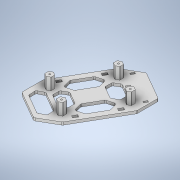
# Autodesk Inventor part: top_body
Saved by Autodesk Inventor 2022 (Build 260153000, 153)
## iProperties
Created: 2022-01-21
Part Number: top_body
Material: Generic
Document SubType Name: Modeling
Designer: felix
Density: 1 g/cm^3
Appearance: Default
Author: felix
Autodesk Inventor part; units mm, degrees
ref_plane "YZ Plane" through (0, 0, 0) normal (1, 0, 0) x (0, 1, 0)
ref_plane "XZ Plane" through (0, 0, 0) normal (0, 1, 0) x (-1, 0, 0)
ref_plane "XY Plane" through (0, 0, 0) normal (0, 0, 1) x (1, 0, 0)
sketch "Sketch1" plane through (0, 0, 0) normal (0, 1, 0) x (-1, 0, 0)
  line L0 (-6.75, 41.286) -> (6.75, 41.286)
  line L1 (-8.75, 41.286) -> (-12.4595, 41.286)
  line L2 (10.832, 42.286) -> (27.4333, 71.0403)
  line L3 (39.1324, 45.1163) -> (-87.7037, 118.3452) construction
  line L4 (27.4333, 73.0403) -> (16.6536, 91.7113)
  line L5 (-8.3049, 49.4102) -> (11.6951, 84.0512) construction
  line L6 (11.6951, 84.0512) -> (-40.2664, 114.0512) construction
  line L7 (-40.2664, 114.0512) -> (-60.2664, 79.4102) construction
  line L8 (-60.2664, 79.4102) -> (-8.3049, 49.4102) construction
  line L9 (27.4333, 73.0403) -> (16.6536, 91.7113)
  line L10 (-13.4595, 41.554) -> (-38.9761, 56.286)
  line L11 (15.9215, 92.4434) -> (-9.5951, 107.1754)
  line L12 (-38.9761, 56.286) -> (-9.5951, 107.1754) construction
  line L13 (8.75, 41.286) -> (9.0999, 41.286)
  line L14 (6.75, 41.286) -> (8.75, 41.286)
  line L15 (-6.75, 41.286) -> (-8.75, 41.286)
  line L16 (-68.0796, 76.6947) -> (-74.8296, 88.386)
  line L17 (-67.0796, 74.9626) -> (-65.2248, 71.7501)
  line L18 (-76.0045, 92.4211) -> (-59.413, 121.1585)
  line L19 (-57.6825, 122.1585) -> (-36.1133, 122.1754)
  line L20 (-57.6825, 122.1585) -> (-36.1133, 122.1754)
  line L21 (-64.4928, 71.0181) -> (-38.9761, 56.286)
  line L22 (-35.1118, 121.9075) -> (-9.5951, 107.1754)
  line L23 (-75.8296, 90.1181) -> (-76.0045, 90.4211)
  line L24 (-74.8296, 88.386) -> (-75.8296, 90.1181)
  line L25 (-68.0796, 76.6947) -> (-67.0796, 74.9626)
  line L26 (-41.8469, 122.123) -> (-39.8469, 122.123)
  line L27 (8.342, 47.7751) -> (2.3676, 47.4271)
  line L28 (0.464, 48.5261) -> (-2.2218, 53.8742)
  line L29 (-2.1666, 55.7718) -> (9.255, 75.5546)
  line L30 (10.8707, 76.5512) -> (16.8452, 76.8992)
  line L31 (18.7488, 75.8002) -> (21.4346, 70.4522)
  line L32 (21.3794, 68.5546) -> (9.9577, 48.7718)
  line L33 (-53.2274, 80.0021) -> (-54.9595, 77.0021)
  line L34 (-55.3925, 76.7521) -> (-58.8566, 76.7521)
  line L35 (-59.2896, 77.0021) -> (-61.0216, 80.0021)
  line L36 (-61.0216, 80.5021) -> (-59.2896, 83.5021)
  line L37 (-58.8566, 83.7521) -> (-55.3925, 83.7521)
  line L38 (-54.9595, 83.5021) -> (-53.2274, 80.5021)
  circle A0 centre (-57.1245, 80.2521) radius 0.9
  line L39 (-37.2595, 107.6594) -> (-35.5274, 110.6594)
  line L40 (-35.5274, 111.1594) -> (-37.2595, 114.1594)
  line L41 (-37.6925, 114.4094) -> (-41.1566, 114.4094)
  line L42 (-41.5896, 114.1594) -> (-43.3216, 111.1594)
  line L43 (-43.3216, 110.6594) -> (-41.5896, 107.6594)
  line L44 (-41.1566, 107.4094) -> (-37.6925, 107.4094)
  circle A1 centre (-39.4245, 110.9094) radius 0.9
  line L45 (-11.3118, 55.8021) -> (-13.0438, 52.8021)
  line L46 (-13.0438, 52.3021) -> (-11.3118, 49.3021)
  line L47 (-10.8788, 49.0521) -> (-7.4147, 49.0521)
  line L48 (-6.9816, 49.3021) -> (-5.2496, 52.3021)
  line L49 (-5.2496, 52.8021) -> (-6.9816, 55.8021)
  line L50 (-7.4147, 56.0521) -> (-10.8788, 56.0521)
  circle A2 centre (-9.1467, 52.5521) radius 0.9
  line L51 (10.7184, 86.4594) -> (12.4504, 83.4594)
  line L52 (6.8212, 86.7094) -> (10.2853, 86.7094)
  line L53 (4.6562, 83.4594) -> (6.3882, 86.4594)
  circle A3 centre (8.5533, 83.2094) radius 0.9
  line L54 (12.4504, 82.9594) -> (10.7184, 79.9594)
  line L55 (10.2853, 79.7094) -> (6.8212, 79.7094)
  line L56 (6.3882, 79.9594) -> (4.6562, 82.9594)
  line L57 (-55.4722, 69.7141) -> (-53.9722, 72.3121)
  line L58 (-53.9722, 72.3121) -> (-49.642, 69.8121)
  line L59 (-49.642, 69.8121) -> (-51.142, 67.2141)
  line L60 (-51.142, 67.2141) -> (-55.4722, 69.7141)
  line L61 (-29.4722, 114.7474) -> (-30.9722, 112.1493)
  line L62 (-30.9722, 112.1493) -> (-26.642, 109.6493)
  line L63 (-26.642, 109.6493) -> (-25.142, 112.2474)
  line L64 (-25.142, 112.2474) -> (-29.4722, 114.7474)
  line L65 (-19.0991, 48.7141) -> (-17.5991, 51.3121)
  line L66 (-17.5991, 51.3121) -> (-21.9292, 53.8121)
  line L67 (-21.9292, 53.8121) -> (-23.4292, 51.2141)
  line L68 (-23.4292, 51.2141) -> (-19.0991, 48.7141)
  line L69 (2.5708, 96.2474) -> (6.9009, 93.7474)
  line L70 (1.0708, 93.6493) -> (2.5708, 96.2474)
  line L71 (5.4009, 91.1493) -> (1.0708, 93.6493)
  line L72 (6.9009, 93.7474) -> (5.4009, 91.1493)
  line L73 (-46.6809, 74.1125) -> (-44.8508, 67.2824)
  line L74 (-43.9189, 66.068) -> (-28.0333, 56.8964)
  line L75 (-26.5157, 56.6966) -> (-19.6855, 58.5267)
  line L76 (-18.2713, 60.9762) -> (-20.1015, 67.8063)
  line L77 (-21.0333, 69.0207) -> (-36.9189, 78.1923)
  line L78 (-38.4366, 78.3921) -> (-45.2667, 76.562)
  line L79 (18.1584, 76.9758) -> (1.0543, 47.3506) construction
  line L80 (-47.6364, 61.286) -> (-30.8723, 90.3222) construction
  line L81 (-30.3159, 51.286) -> (-13.5518, 80.3222) construction
  line L82 (12.8814, 45.8357) -> (-2.7058, 54.8379) construction
  line L83 (25.3698, 67.436) -> (9.8848, 76.3791) construction
  line L84 (-28.8857, 104.9347) -> (-22.0556, 106.7649)
  line L85 (-20.5379, 106.5651) -> (-4.6523, 97.3935)
  line L86 (-3.7204, 96.1791) -> (-1.8903, 89.3489)
  line L87 (-3.3045, 86.8995) -> (-10.1347, 85.0693)
  line L88 (-11.6523, 85.2691) -> (-27.5379, 94.4407)
  line L89 (-28.4698, 95.6551) -> (-30.2999, 102.4852)
  line L90 (-18.2554, 112.1754) -> (-35.0194, 83.1393) construction
  line L91 (-0.9349, 102.1754) -> (-17.6989, 73.1393) construction
  line L92 (-57.1245, 80.2521) -> (8.5533, 83.2094) construction
  line L93 (-9.1467, 52.5521) -> (-39.4245, 110.9094) construction
  line L94 (-17.7537, 59.0444) -> (-47.1986, 76.0444) construction
  line L95 (-1.3727, 87.4171) -> (-30.8175, 104.4171) construction
  line L96 (-52.6513, 88.8701) -> (-40.527, 81.8701) construction
  line L97 (-44.6513, 102.7265) -> (-32.527, 95.7265) construction
  line L98 (-36.6202, 102.6368) -> (-48.5581, 81.9597) construction
  line L99 (3.4953, 73.5784) -> (-3.3351, 61.7479)
  line L100 (-5.0895, 60.748) -> (-10.826, 60.8121)
  line L101 (-12.5244, 61.7927) -> (-15.4482, 66.7286)
  line L102 (-15.4595, 68.7479) -> (-8.6291, 80.5784)
  line L103 (-6.8747, 81.5783) -> (-1.1382, 81.5143)
  line L104 (0.5603, 80.5337) -> (3.484, 75.5977)
  line L105 (-3.9199, 60.735) -> (-16.0443, 67.735) construction
  line L106 (4.0801, 74.5914) -> (-8.0443, 81.5914) construction
  line L107 (-0.0131, 81.5017) -> (-11.951, 60.8247) construction
  arc A4 (-57.6825, 122.1585) -> (-59.413, 121.1585) centre (-57.681, 120.1585) ccw
  arc A5 (-76.0045, 92.4211) -> (-76.0045, 90.4211) centre (-74.2725, 91.4211) ccw
  arc A6 (-35.1118, 121.9075) -> (-36.1133, 122.1754) centre (-36.1118, 120.1754) ccw
  arc A7 (16.6536, 91.7113) -> (15.9215, 92.4434) centre (14.9215, 90.7113) ccw
  arc A8 (27.4333, 71.0403) -> (27.4333, 73.0403) centre (25.7012, 72.0403) ccw
  arc A9 (9.0999, 41.286) -> (10.832, 42.286) centre (9.0999, 43.286) ccw
  arc A10 (-13.4595, 41.554) -> (-12.4595, 41.286) centre (-12.4595, 43.286) ccw
  arc A11 (-65.2248, 71.7501) -> (-64.4928, 71.0181) centre (-63.4928, 72.7501) ccw
  arc A12 (-61.0216, 80.5021) -> (-61.0216, 80.0021) centre (-60.5886, 80.2521) ccw
  arc A13 (-58.8566, 83.7521) -> (-59.2896, 83.5021) centre (-58.8566, 83.2521) ccw
  arc A14 (-54.9595, 83.5021) -> (-55.3925, 83.7521) centre (-55.3925, 83.2521) ccw
  arc A15 (-53.2274, 80.0021) -> (-53.2274, 80.5021) centre (-53.6604, 80.2521) ccw
  arc A16 (-55.3925, 76.7521) -> (-54.9595, 77.0021) centre (-55.3925, 77.2521) ccw
  arc A17 (-59.2896, 77.0021) -> (-58.8566, 76.7521) centre (-58.8566, 77.2521) ccw
  arc A18 (-43.3216, 111.1594) -> (-43.3216, 110.6594) centre (-42.8886, 110.9094) ccw
  arc A19 (-41.1566, 114.4094) -> (-41.5896, 114.1594) centre (-41.1566, 113.9094) ccw
  arc A20 (-37.2595, 114.1594) -> (-37.6925, 114.4094) centre (-37.6925, 113.9094) ccw
  arc A21 (-35.5274, 110.6594) -> (-35.5274, 111.1594) centre (-35.9604, 110.9094) ccw
  arc A22 (-37.6925, 107.4094) -> (-37.2595, 107.6594) centre (-37.6925, 107.9094) ccw
  arc A23 (-41.5896, 107.6594) -> (-41.1566, 107.4094) centre (-41.1566, 107.9094) ccw
  arc A24 (6.8212, 86.7094) -> (6.3882, 86.4594) centre (6.8212, 86.2094) ccw
  arc A25 (10.7184, 86.4594) -> (10.2853, 86.7094) centre (10.2853, 86.2094) ccw
  arc A26 (12.4504, 82.9594) -> (12.4504, 83.4594) centre (12.0174, 83.2094) ccw
  arc A27 (10.2853, 79.7094) -> (10.7184, 79.9594) centre (10.2853, 80.2094) ccw
  arc A28 (6.3882, 79.9594) -> (6.8212, 79.7094) centre (6.8212, 80.2094) ccw
  arc A29 (4.6562, 83.4594) -> (4.6562, 82.9594) centre (5.0892, 83.2094) ccw
  arc A30 (-13.0438, 52.8021) -> (-13.0438, 52.3021) centre (-12.6108, 52.5521) ccw
  arc A31 (-11.3118, 49.3021) -> (-10.8788, 49.0521) centre (-10.8788, 49.5521) ccw
  arc A32 (-7.4147, 49.0521) -> (-6.9816, 49.3021) centre (-7.4147, 49.5521) ccw
  arc A33 (-5.2496, 52.3021) -> (-5.2496, 52.8021) centre (-5.6826, 52.5521) ccw
  arc A34 (-6.9816, 55.8021) -> (-7.4147, 56.0521) centre (-7.4147, 55.5521) ccw
  arc A35 (-10.8788, 56.0521) -> (-11.3118, 55.8021) centre (-10.8788, 55.5521) ccw
  arc A36 (-45.2667, 76.562) -> (-46.6809, 74.1125) centre (-44.7491, 74.6301) ccw
  arc A37 (-36.9189, 78.1923) -> (-38.4366, 78.3921) centre (-37.9189, 76.4603) ccw
  arc A38 (-44.8508, 67.2824) -> (-43.9189, 66.068) centre (-42.9189, 67.8) ccw
  arc A39 (-28.0333, 56.8964) -> (-26.5157, 56.6966) centre (-27.0333, 58.6284) ccw
  arc A40 (-19.6855, 58.5267) -> (-18.2713, 60.9762) centre (-20.2032, 60.4586) ccw
  arc A41 (-20.1015, 67.8063) -> (-21.0333, 69.0207) centre (-22.0333, 67.2887) ccw
  arc A42 (-28.4698, 95.6551) -> (-27.5379, 94.4407) centre (-26.5379, 96.1728) ccw
  arc A43 (-28.8857, 104.9347) -> (-30.2999, 102.4852) centre (-28.3681, 103.0029) ccw
  arc A44 (-20.5379, 106.5651) -> (-22.0556, 106.7649) centre (-21.5379, 104.833) ccw
  arc A45 (-3.7204, 96.1791) -> (-4.6523, 97.3935) centre (-5.6523, 95.6614) ccw
  arc A46 (-3.3045, 86.8995) -> (-1.8903, 89.3489) centre (-3.8222, 88.8313) ccw
  arc A47 (-11.6523, 85.2691) -> (-10.1347, 85.0693) centre (-10.6523, 87.0012) ccw
  arc A48 (-2.1666, 55.7718) -> (-2.2218, 53.8742) centre (-0.4346, 54.7718) ccw
  arc A49 (10.8707, 76.5512) -> (9.255, 75.5546) centre (10.9871, 74.5546) ccw
  arc A50 (18.7488, 75.8002) -> (16.8452, 76.8992) centre (16.9615, 74.9026) ccw
  arc A51 (21.3794, 68.5546) -> (21.4346, 70.4522) centre (19.6473, 69.5546) ccw
  arc A52 (8.342, 47.7751) -> (9.9577, 48.7718) centre (8.2257, 49.7718) ccw
  arc A53 (0.464, 48.5261) -> (2.3676, 47.4271) centre (2.2512, 49.4237) ccw
  arc A54 (-15.4595, 68.7479) -> (-15.4482, 66.7286) centre (-13.7274, 67.7479) ccw
  arc A55 (-6.8747, 81.5783) -> (-8.6291, 80.5784) centre (-6.897, 79.5784) ccw
  arc A56 (0.5603, 80.5337) -> (-1.1382, 81.5143) centre (-1.1605, 79.5144) ccw
  arc A57 (3.4953, 73.5784) -> (3.484, 75.5977) centre (1.7632, 74.5784) ccw
  arc A58 (-5.0895, 60.748) -> (-3.3351, 61.7479) centre (-5.0671, 62.7479) ccw
  arc A59 (-12.5244, 61.7927) -> (-10.826, 60.8121) centre (-10.8037, 62.812) ccw
  line L108 (-45.2361, 101.7135) -> (-52.0665, 89.883)
  line L109 (-52.0552, 87.8637) -> (-49.1315, 82.9278)
  line L110 (-47.433, 81.9472) -> (-41.6965, 81.8831)
  line L111 (-37.7452, 102.6494) -> (-43.4818, 102.7134)
  line L112 (-33.1231, 96.7328) -> (-36.0468, 101.6688)
  line L113 (-39.9421, 82.883) -> (-33.1118, 94.7135)
  arc A60 (-41.6965, 81.8831) -> (-39.9421, 82.883) centre (-41.6742, 83.883) ccw
  arc A61 (-33.1118, 94.7135) -> (-33.1231, 96.7328) centre (-34.8438, 95.7135) ccw
  arc A62 (-36.0468, 101.6688) -> (-37.7452, 102.6494) centre (-37.7676, 100.6495) ccw
  arc A63 (-43.4818, 102.7134) -> (-45.2361, 101.7135) centre (-43.5041, 100.7135) ccw
  arc A64 (-52.0665, 89.883) -> (-52.0552, 87.8637) centre (-50.3345, 88.883) ccw
  arc A65 (-49.1315, 82.9278) -> (-47.433, 81.9472) centre (-47.4107, 83.9471) ccw
  point P0 (10.2546, 41.286)
  point P1 (-12.9954, 41.286)
  point P2 (28.0107, 72.0403)
  point P3 (19.1326, 56.6632)
  point P4 (-67.7039, 106.7983)
  point P5 (-8.3049, 49.4102)
  point P6 (-24.2856, 81.7307)
  point P7 (9.4185, 47.8379)
  point P8 (21.9185, 69.4885)
  point P9 (-53.0831, 80.2521)
  point P10 (-55.1038, 76.7521)
  point P11 (-59.1452, 76.7521)
  point P12 (-61.166, 80.2521)
  point P13 (-59.1452, 83.7521)
  point P14 (-55.1038, 83.7521)
  point P15 (-37.4038, 107.4094)
  point P16 (-35.3831, 110.9094)
  point P17 (-37.4038, 114.4094)
  point P18 (-41.4452, 114.4094)
  point P19 (-43.466, 110.9094)
  point P20 (-41.4452, 107.4094)
  point P21 (-11.1674, 56.0521)
  point P22 (-13.1882, 52.5521)
  point P23 (-11.1674, 49.0521)
  point P24 (-7.126, 49.0521)
  point P25 (-5.1053, 52.5521)
  point P26 (-7.126, 56.0521)
  point P27 (10.574, 86.7094)
  point P28 (12.5947, 83.2094)
  point P29 (6.5326, 86.7094)
  point P30 (4.5118, 83.2094)
  point P31 (10.574, 79.7094)
  point P32 (6.5326, 79.7094)
  point P33 (-44.6364, 66.4822)
  point P34 (-27.3159, 56.4822)
  point P35 (-20.3159, 68.6065)
  point P36 (-37.6364, 78.6065)
  point P37 (-21.2554, 106.9793)
  point P38 (-3.9349, 96.9793)
  point P39 (-10.9349, 84.8549)
  point P40 (-28.2554, 94.8549)
  point P41 (8.5533, 83.2094)
  dimension "d82" = 23.25
  dimension "d88" = 120
  dimension "d89" = 120
  dimension "d90" = 35.512
  dimension "d91" = 17.756
  dimension "d92" = 17.756
  dimension "d95" = 40
  dimension "d97" = 20
  dimension "d99" = 30
  dimension "d102" = 60
  dimension "d145" = 180
  dimension "d146" = 30
  dimension "d147" = 8.1242
  dimension "d148" = 8.1242
  dimension "d155" = 1.8
  dimension "d156" = 7
  dimension "d157" = 1.4
  dimension "d158" = 1.4
  dimension "d160" = 3
  dimension "d162" = 3
  dimension "d163" = 9
  dimension "d169" = 6
  dimension "d170" = 10
  dimension "d171" = 20
  dimension "d172" = 14
  dimension "d179" = 7
  dimension "d181" = 2
  dimension "d186" = 0.5
  dimension "d187" = 0.5
  dimension "d189" = 2
  dimension "d190" = 2
  dimension "d191" = 4
  dimension "d192" = 16
  dimension "d193" = 8
  dimension "d194" = 14
  dimension "d195" = 8
  dimension "d204" = 14
  dimension "d206" = 18.762
  dimension "d207" = 28.2702
  dimension "d238" = 5
  dimension "d244" = 25
  dimension "d245" = 12.5
  dimension "d246" = 0
  dimension "d247" = 4
  constraints: 228 end point, 124 point on circle, 112 tangent, 110 point on line, 79 symmetric about line, 66 centre point, 51 equal radius, 16 parallel, 9 equal length, 6 perpendicular, 4 collinear, 3 coincident, 3 midpoint, 2 horizontal, 22 other
  measures "d82" distance of point (10.255, 41.286) point (-12.995, 41.286)
  measures "d88" angle of L2 L1
  measures "d89" angle of L4 L2
  measures "d90" distance of point (10.255, 41.286) point (28.011, 72.04)
  measures "d91" distance of point (19.133, 56.663) point (10.255, 41.286)
  measures "d92" distance of point (28.011, 72.04) point (19.133, 56.663)
  measures "d95" distance of L5.start L5.end
  measures "d97" distance from line of L3 L5.start
  measures "d99" distance of L10.end point (-12.995, 41.286)
  measures "d102" distance of L7.end L5.start
  measures "d145" angle of L10 L21
  measures "d146" distance from line of L5 point (-24.286, 81.731)
  measures "d147" distance from line of L0 L5.start
  measures "d148" distance from line of L4 L5.end
  measures "d155" diameter of A0
  measures "d156" distance between parallel lines of L38 L35
  measures "d157" distance edge to line of A0 L7
  measures "d158" distance edge to line of A0 L8
  measures "d160" distance between parallel lines of L58 L60
  measures "d162" distance between parallel lines of L8 L58
  measures "d163" distance between parallel lines of L57 L7
  measures "d169" distance between parallel lines of L21 L74
  measures "d170" distance from line of L12 point (-27.316, 56.482)
  measures "d171" distance of point (-44.636, 66.482) point (-27.316, 56.482)
  measures "d172" distance between parallel lines of L77 L74
  measures "d179" distance from line of L94.end L80
  measures "d181" radius of A4
  measures "d186" radius of A12
  measures "d187" radius of A27
  measures "d189" radius of A36
  measures "d190" radius of A54
  measures "d191" distance between parallel lines of L29 L99
  measures "d192" distance of L105.start L106.start
  measures "d193" distance from line of L3 L106.start
  measures "d194" distance between parallel lines of L99 L102
  measures "d195" distance between parallel lines of L106 L3
  measures "d204" distance between parallel lines of L32 L29
  measures "d206" distance between parallel lines of L88 L77
  measures "d207" distance between parallel lines of L113 L102
  measures "d238" distance of L59.end L57.start
  measures "d244" distance of point (21.919, 69.488) point (9.419, 47.838)
  measures "d245" distance from line of L3 point (9.419, 47.838)
  measures "d246" angle of L83 L82
  measures "d247" distance between parallel lines of L2 L32
extrude "Extrusion1_main_body" add sketch "Sketch1" along normal blind 3 contours L15 L1 A10 L10 L21 A11 L17 L25 L16 L24 L23 A5 L18 A4 L19 A6 L22 L11 A7 L4 A8 L2 A9 L13 L14 L0
extrude "Extrusion2_main_body" add sketch "Sketch1" along normal blind 16 contours L33 A16 L34 A17 L35 A12 L36 A13 L37 A14 L38 A15 | A22 L44 A23 L43 A18 L42 A19 L41 A20 L40 A21 L39 | A35 L50 A34 L49 A33 L48 A32 L47 A31 L46 A30 L45 | L51 A26 L54 A27 L55 A28 L56 A29 L53 A24 L52 A25
extrude "Extrusion3_main_body" add sketch "Sketch1" along normal blind 13 contours A0 | A1 | A2 | A3
sketch "Sketch2_insert" plane through (0, 0, 0) normal (0, -1, 0) x (1, 0, 0)
  line L0 (43.2184, 119.2084) -> (66.2184, 79.3712)
  line L1 (66.2184, 79.3712) -> (65.006, 78.6712)
  line L2 (65.006, 78.6712) -> (42.006, 118.5084)
  line L3 (42.006, 118.5084) -> (43.2184, 119.2084)
  line L4 (59.413, 121.1585) -> (76.0045, 92.4211) projected
  line L5 (52.0665, 89.883) -> (45.2361, 101.7135) projected
  line L6 (64.4928, 71.0181) -> (13.4595, 41.554) projected
  line L7 (-15.9215, 92.4434) -> (35.1118, 121.9075) projected
  line L8 (66.7328, 106.2263) -> (52.4033, 97.9531) construction
  line L9 (59.413, 121.1585) -> (76.0045, 92.4211) projected
  line L10 (51.006, 102.9199) -> (47.5419, 100.9199)
  line L11 (47.5419, 100.9199) -> (52.5419, 92.2597)
  line L12 (52.5419, 92.2597) -> (56.006, 94.2597)
  line L13 (52.2184, 103.6199) -> (53.9504, 104.6199)
  line L14 (53.9504, 104.6199) -> (58.9504, 95.9597)
  line L15 (58.9504, 95.9597) -> (57.2184, 94.9597)
  line L16 (46.5335, 118.4665) -> (49.9976, 120.4665)
  line L17 (49.9976, 120.4665) -> (50.9976, 118.7345)
  line L18 (50.9976, 118.7345) -> (47.5335, 116.7345)
  line L19 (47.5335, 116.7345) -> (46.5335, 118.4665)
  line L20 (36.1133, 122.1754) -> (57.6825, 122.1585) projected
  line L21 (67.2335, 82.6131) -> (70.6976, 84.6131)
  line L22 (70.6976, 84.6131) -> (69.6976, 86.3451)
  line L23 (69.6976, 86.3451) -> (66.2335, 84.3451)
  line L24 (66.2335, 84.3451) -> (67.2335, 82.6131)
  point P0 (0, 0)
  point P1 (54.7184, 99.2898)
  point P2 (67.7088, 106.7898)
  point P3 (50.0419, 96.5898)
  dimension "d249" = 1.4
  dimension "d250" = 15
  dimension "d251" = 46
  dimension "d252" = 23
  dimension "d254" = 10
  dimension "d255" = 4
  dimension "d256" = 1.6
  dimension "d257" = 10
  dimension "d258" = 2
  dimension "d265" = 4
  dimension "d266" = 2
  dimension "d267" = 2.5
  dimension "d268" = 2.3
  dimension "d269" = 1.698
  constraints: 38 end point, 12 parallel, 7 point on line, 6 perpendicular, 4 symmetric about line, 3 midpoint
  measures "d249" distance of L2.end L0.start
  measures "d250" distance between parallel lines of L4 L0
  measures "d251" distance of L0.start L0.end
  measures "d252" distance of L0.start point (54.718, 99.29)
  measures "d254" distance between parallel lines of L12 L10
  measures "d255" distance of L11.end L12.end
  measures "d256" distance between parallel lines of L5 L11
  measures "d257" distance of L13.end L14.end
  measures "d258" distance of L13.start L13.end
  measures "d265" distance of L16.start L16.end
  measures "d266" distance between parallel lines of L18 L16
  measures "d267" distance between parallel lines of L0 L19
  measures "d268" distance between parallel lines of L16 L3
  measures "d269" distance from line of L16.end L20
extrude "Extrusion1_feature1" cut sketch "Sketch2_insert" against normal blind 1.5 contours L0 L1 L2 L3
extrude "Extrusion2_feature1" cut sketch "Sketch2_insert" against normal blind 1.2 contours L13 L14 L15 L0
extrude "Extrusion3_feature1" cut sketch "Sketch2_insert" against normal blind 3 contours L2 L12 L11 L10
extrude "Extrusion4_feature1_zip_ties" cut sketch "Sketch2_insert" against normal blind 3 contours L16 L17 L18 L19 | L24 L23 L22 L21
body "Solid1"
